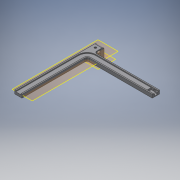
# Autodesk Inventor part: Top Clip
Saved by Autodesk Inventor 2017 (Build 210142000, 142)
## iProperties
Created: 2017-03-25
Part Number: Top Clip
Material: Generic
Document SubType Name: Modeling
Designer: Diego
Density: 1 g/cm^3
Appearance: Default
Author: Diego
Autodesk Inventor part; units mm, degrees
ref_plane "YZ Plane" through (0, 0, 0) normal (1, 0, 0) x (0, 1, 0)
ref_plane "XZ Plane" through (0, 0, 0) normal (0, 1, 0) x (-1, 0, 0)
ref_plane "XY Plane" through (0, 0, 0) normal (0, 0, 1) x (1, 0, 0)
sketch "Sketch1" plane through (0, 0, 0) normal (1, 0, 0) x (0, 1, 0)
  line L0 (67.2039, 7.058) -> (87.2039, 7.058)
  line L1 (87.2039, 7.058) -> (87.2039, 31.058)
  line L2 (87.2039, 31.058) -> (-82.7961, 31.058)
  line L3 (-82.7961, 31.058) -> (-82.7961, 24.058)
  line L4 (-82.7961, 24.058) -> (80.2039, 24.058)
  line L5 (80.2039, 24.058) -> (80.2039, 14.058)
  line L6 (80.2039, 14.058) -> (67.2039, 14.058)
  line L7 (67.2039, 14.058) -> (67.2039, 7.058)
  dimension "d0" = 10
  dimension "d1" = 13
  dimension "d2" = 7
  dimension "d3" = 7
  dimension "d5" = 7
  dimension "d6" = 170
  constraints: 16 end point, 6 perpendicular, 1 horizontal, 1 vertical
  measures "d0" distance between parallel lines of L6 L4
  measures "d1" distance between parallel lines of L7 L5
  measures "d2" distance between parallel lines of L1 L5
  measures "d3" distance between parallel lines of L0 L6
  measures "d5" distance between parallel lines of L4 L2
  measures "d6" distance between parallel lines of L1 L3
extrude "Extrusion1" add sketch "Sketch1" along normal blind 15
sketch "Sketch2" plane through (15, 0, 0) normal (1, 0, 0) x (0, 0, -1)
  line L0 (-7.058, 67.2039) -> (-7.058, 87.2039) projected
  line L1 (-7.058, 87.2039) -> (-31.058, 87.2039) projected
  line L2 (-31.058, 87.2039) -> (-31.058, -82.7961) projected
  line L3 (-31.058, -82.7961) -> (-24.058, -82.7961) projected
  line L4 (-24.058, -82.7961) -> (-24.058, 80.2039) projected
  line L5 (-24.058, 80.2039) -> (-14.058, 80.2039) projected
  line L6 (-14.058, 80.2039) -> (-14.058, 67.2039) projected
  line L7 (-14.058, 67.2039) -> (-7.058, 67.2039) projected
  line L8 (-31.058, 52.2039) -> (-24.058, 52.2039)
  line L9 (-24.058, 80.2039) -> (-24.058, -82.7961) projected
  line L10 (-24.058, 67.2039) -> (-31.058, 67.2039)
  point P0 (0, 0)
  dimension "d9" = 15
  dimension "d10" = 20
  constraints: 4 end point, 4 point on line, 1 parallel, 1 perpendicular
  measures "d9" distance between parallel lines of L10 L8
  measures "d10" distance between parallel lines of L1 L10
extrude "Extrusion2" add sketch "Sketch2" along normal blind 135 contours L10 L4 L8 L2
fillet "Fillet1" radius 5 2 edges at (15, 67.2039, 27.558) (15, 52.2039, 27.558)
ref_plane "Work Plane1" through (0, 67.2039, 10.558) normal (0, 0, 1) x (1, 0, 0)
sketch "Sketch6" plane through (150, 0, 0) normal (1, 0, 0) x (0, 0, -1)
  line L0 (-31.058, 52.2039) -> (-24.058, 52.2039) projected
  line L1 (-24.058, 52.2039) -> (-24.058, 67.2039) projected
  line L2 (-24.058, 67.2039) -> (-31.058, 67.2039) projected
  line L3 (-31.058, 67.2039) -> (-31.058, 52.2039) projected
  line L4 (-31.058, 54.4039) -> (-29.058, 54.4039)
  line L5 (-29.058, 54.4039) -> (-29.058, 65.0039)
  line L6 (-29.058, 65.0039) -> (-31.058, 65.0039)
  line L7 (-31.058, 67.2039) -> (-31.058, 52.2039) construction
  line L8 (-31.058, 59.7039) -> (-29.058, 59.7039) construction
  point P0 (0, 0)
  dimension "d23" = 10.6
  dimension "d24" = 2
  constraints: 8 end point, 3 perpendicular, 2 midpoint, 2 point on line, 1 horizontal
  measures "d23" distance between parallel lines of L4 L6
  measures "d24" distance between parallel lines of L5 L3
sketch "Sketch7" plane through (0, -82.7961, 31.058) normal (0, 0, 1) x (1, 0, 0)
  line L0 (0, 0) -> (0, 170) projected
  line L1 (0, 0) -> (15, 0) projected
  line L2 (15, 130) -> (15, 0) projected
  arc A0 (20, 135) -> (15, 130) centre (20, 130) ccw projected
  line L3 (20, 135) -> (150, 135) projected
  line L4 (150, 150) -> (150, 135) projected
  line L5 (20, 150) -> (150, 150) projected
  arc A1 (15, 155) -> (20, 150) centre (20, 155) ccw projected
  line L6 (15, 170) -> (15, 155) projected
  line L7 (0, 170) -> (15, 170) projected
  arc A2 (20, 142.5) -> (7.5, 130) centre (20, 130) ccw
  line L8 (150, 135) -> (150, 150) projected
  line L9 (150, 142.5) -> (20, 142.5)
  line L10 (0, 0) -> (15, 0) projected
  line L11 (7.5, 0) -> (7.5, 130)
  point P0 (0, 82.7961)
  dimension "d25" = 7.5
  constraints: 4 end point, 2 midpoint, 2 point on circle, 1 centre point, 1 parallel, 1 perpendicular
  measures "d25" radial gap between concentric circles of A2 A0
sweep "Sweep1" cut profiles "Sketch6" path "Sketch7" path curves L9 A2 L11 contours L3 L6 L5 L4
sketch "Sketch8" plane through (0, -82.7961, 31.058) normal (0, 0, 1) x (1, 0, 0)
  line L0 (150, 147.8) -> (150, 137.2) projected
  line L1 (150, 147.8) -> (20, 147.8) projected
  arc A0 (20, 147.8) -> (2.2, 130) centre (20, 130) ccw projected
  line L2 (2.2, 130) -> (2.2, 0) projected
  line L3 (12.8, 0) -> (2.2, 0) projected
  line L4 (12.8, 130) -> (12.8, 0) projected
  arc A1 (20, 137.2) -> (12.8, 130) centre (20, 130) ccw projected
  line L5 (150, 137.2) -> (20, 137.2) projected
  line L6 (2.2, 0) -> (2.2, 130) projected
  arc A2 (20, 147.8) -> (2.2, 130) centre (20, 130) ccw projected
  line L7 (20, 147.8) -> (150, 147.8) projected
  line L8 (150, 150) -> (150, 147.8) projected
  line L9 (20, 150) -> (150, 150) projected
  arc A3 (15, 155) -> (20, 150) centre (20, 155) ccw projected
  line L10 (15, 170) -> (15, 155) projected
  line L11 (0, 170) -> (15, 170) projected
  line L12 (0, 0) -> (0, 170) projected
  line L13 (0, 0) -> (2.2, 0) projected
  line L14 (12.8, 130) -> (12.8, 0) projected
  line L15 (12.8, 0) -> (15, 0) projected
  line L16 (15, 130) -> (15, 0) projected
  arc A4 (20, 135) -> (15, 130) centre (20, 130) ccw projected
  line L17 (20, 135) -> (150, 135) projected
  line L18 (150, 137.2) -> (150, 135) projected
  line L19 (150, 137.2) -> (20, 137.2) projected
  arc A5 (20, 137.2) -> (12.8, 130) centre (20, 130) ccw projected
  line L20 (150, 135) -> (150, 150) projected
  line L21 (150, 142.5) -> (135.884, 142.5) construction
  line L22 (150, 145) -> (140, 147.8)
  line L23 (150, 147.8) -> (20, 147.8) construction
  line L24 (140, 147.8) -> (135, 147.8)
  line L25 (135, 147.8) -> (135, 137.2)
  line L26 (150, 137.2) -> (20, 137.2) projected
  line L27 (135, 137.2) -> (140, 137.2)
  line L28 (150, 140) -> (140, 137.2)
  line L29 (150, 140) -> (150, 145) construction
  line L30 (150, 145) -> (150, 140)
  point P0 (0, 82.7961)
  dimension "d29" = 5
  dimension "d30" = 5
  dimension "d31" = 15
  dimension "d32" = 5
  constraints: 16 end point, 5 point on line, 2 collinear, 2 midpoint, 1 horizontal, 1 perpendicular, 1 vertical
  measures "d29" distance of L22.end L24.end
  measures "d30" distance of L25.end L27.end
  measures "d31" distance between parallel lines of L0 L25
  measures "d32" distance of L28.start L22.start
extrude "Extrusion5" cut sketch "Sketch8" against normal blind 5.75 contours L0 L28 L5 L25 L1 L22
fillet "Fillet2" radius 4 2 edges at (7.5, 87.2039, 31.058) (7.5, 87.2039, 7.058)
fillet "Fillet3" radius 2 2 edges at (7.5, 80.2039, 24.058) (7.5, 80.2039, 14.058)
fillet "Fillet4" radius 2 2 edges at (7.5, 67.2039, 7.058) (7.5, 67.2039, 14.058)
sketch "Sketch9" plane through (20, 67.2039, 31.058) normal (0, 0, 1) x (1, 0, 0)
  line L0 (-20, 16) -> (-5, 16) projected
  line L1 (-5, 16) -> (-5, 5) projected
  circle A0 centre (-12.5, 9.6858) radius 2.175
  line L2 (-12.5, 16) -> (-12.5, 9.6858) construction
  line L3 (-5, 9.6858) -> (-12.5, 9.6858) construction
  point P0 (-20, -67.2039)
  dimension "d38" = 4.35
  dimension "d39" = 6.3142
  constraints: 4 end point, 1 centre point, 1 coincident, 1 horizontal, 1 midpoint, 1 point on line, 1 vertical
  measures "d38" diameter of A0
  measures "d39" distance between parallel lines of L0 L3
extrude "Extrusion6" cut sketch "Sketch9" against normal blind 10
ref_plane "Work Plane2" through (20, 67.2039, 27.558) normal (0, 0, 1) x (1, 0, 0)
sketch "Sketch10" plane through (20, 67.2039, 27.558) normal (0, 0, 1) x (1, 0, 0)
  line L0 (-14.2331, 11) -> (-20, 11) projected
  line L1 (-20, 11) -> (-20, 13) projected
  line L2 (-20, 13) -> (-5, 13) projected
  line L3 (-5, 13) -> (-5, 11) projected
  line L4 (-5, 11) -> (-10.7669, 11) projected
  arc A0 (-14.2331, 11) -> (-10.7669, 11) centre (-12.5, 9.6858) ccw projected
  line L5 (-5, 11) -> (-10.7669, 11) projected
  line L6 (-5, 5) -> (-5, 11) projected
  arc A1 (-5, 5) -> (0, 0) centre (0, 5) ccw projected
  line L7 (0, 0) -> (130, 0) projected
  line L8 (130, -15) -> (130, 0) projected
  line L9 (130, -15) -> (0, -15) projected
  arc A2 (0, -15) -> (-5, -20) centre (0, -20) ccw projected
  line L10 (-5, -150) -> (-5, -20) projected
  line L11 (-20, -150) -> (-5, -150) projected
  line L12 (-20, 11) -> (-20, -150) projected
  line L13 (-14.2331, 11) -> (-20, 11) projected
  line L14 (-10.4071, 6.0608) -> (-14.5929, 6.0608)
  line L15 (-14.5929, 6.0608) -> (-16.6858, 9.6858)
  line L16 (-16.6858, 9.6858) -> (-14.5929, 13.3108)
  line L17 (-14.5929, 13.3108) -> (-10.4071, 13.3108)
  line L18 (-8.3142, 9.6858) -> (-12.5, 9.6858) construction
  line L19 (-10.4071, 13.3108) -> (-5, 13.3108)
  line L20 (-5, 2) -> (-5, 16) projected
  line L21 (-10.4071, 6.0608) -> (-5, 6.0608)
  line L22 (-5, 6.0608) -> (-5, 13.3108)
  line L23 (-10.4071, 13.3108) -> (-10.372, 13)
  point P0 (-20, -67.2039)
  dimension "d42" = 7.25
  constraints: 18 end point, 3 point on line, 2 horizontal, 1 coincident, 1 collinear, 1 horizontal alignment, 1 parallel, 10 other
  measures "d42" distance between parallel lines of L14 L17
extrude "Extrusion7" cut sketch "Sketch10" along normal mid plane 4 contours A0 L4 L6 L21 L14 L15 L16 L0 | L0 L16 L2 L3 L4 A0 | L16 L17 L23 L2 | L23 L19 L20 L2
equation "\"d3\" = d2"
equation "\"d5\" = d2"
equation "\"d30\" = d29"
body "Solid1"
